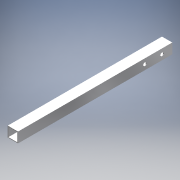
# Autodesk Inventor part: bar for front wepaon
Saved by Autodesk Inventor 2019 (Build 230136000, 136)
## iProperties
Created: 2017-12-10
Part Number: bar for front wepaon
Material: Aluminum 6061
Document SubType Name: Modeling
Designer: rk_fe
Density: 2.7 g/cm^3
Appearance: Aluminum - Flat
Author: rk_fe
Autodesk Inventor part; units mm, degrees
ref_plane "YZ Plane" through (0, 0, 0) normal (1, 0, 0) x (0, 1, 0)
ref_plane "XZ Plane" through (0, 0, 0) normal (0, 1, 0) x (-1, 0, 0)
ref_plane "XY Plane" through (0, 0, 0) normal (0, 0, 1) x (1, 0, 0)
sketch "Sketch1" plane through (0, 0, 0) normal (0, 0, 1) x (1, 0, 0)
  line L0 (0, 0) -> (25.4, 0)
  line L1 (25.4, 0) -> (25.4, 25.4)
  line L2 (25.4, 25.4) -> (0, 25.4)
  line L3 (0, 25.4) -> (0, 0)
  dimension "d0" = 25.4
  dimension "d1" = 25.4
  constraints: 8 end point, 2 parallel, 1 horizontal, 1 perpendicular
  measures "d0" distance of L0.end L1.end
  measures "d1" distance of L1.end L2.end
extrude "Extrusion1" add sketch "Sketch1" along normal blind 381
sketch "Sketch2" plane through (0, 0, 381) normal (0, 0, 1) x (1, 0, 0)
  line L0 (25.4, 25.4) -> (0, 25.4) projected
  line L1 (0, 0) -> (25.4, 0) projected
  line L2 (0, 25.4) -> (25.4, 0)
  line L3 (25.4, 25.4) -> (0, 0)
  line L4 (1.5875, 1.5875) -> (23.8125, 1.5875)
  line L5 (23.8125, 1.5875) -> (23.8125, 23.8125)
  line L6 (23.8125, 23.8125) -> (1.5875, 23.8125)
  line L7 (1.5875, 23.8125) -> (1.5875, 1.5875)
  dimension "d4" = 1.5875
  dimension "d5" = 1.5875
  constraints: 12 end point, 2 parallel, 2 point on line, 1 horizontal, 1 perpendicular
  measures "d4" distance between parallel lines of L0 L6
  measures "d5" distance between parallel lines of L1 L4
extrude "Extrusion2" cut sketch "Sketch2" against normal blind 436.88 contours L5 L2 L3 | L3 L2 L6 | L2 L3 L7 | L2 L4 L3
sketch "Sketch4" plane through (25.4, 0, 0) normal (1, 0, 0) x (0, 0, -1)
  line L0 (0, 1.5875) -> (0, 23.8125) projected
  line L1 (0, 12.7) -> (-101.6, 12.7)
  circle A0 centre (-67.7333, 12.7) radius 4.064
  circle A1 centre (-25.4, 12.7) radius 4.064
  point P0 (0, 0)
  dimension "d14" = 101.6
  dimension "d15" = 33.8667
  dimension "d16" = 76.2
  dimension "d17" = 8.128
  dimension "d18" = 8.128
  constraints: 2 centre point, 2 end point, 2 point on line, 1 horizontal, 1 midpoint
  measures "d14" distance of L1.start L1.end
  measures "d15" distance of L1.end A0.centre
  measures "d16" distance of L1.end A1.centre
  measures "d17" diameter of A1
  measures "d18" diameter of A0
extrude "Extrusion4" cut sketch "Sketch4" against normal blind 25.4
body "Solid1"
